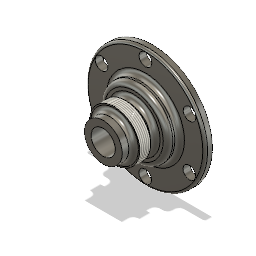
615789d2-998c-4c85-b917-ce7dc0a0639c (Autodesk Fusion 360 design; units mm, degrees)
Autodesk Fusion 360 part; units mm, degrees
sketch "Sketch1" plane through (0, 0, 0) normal (0, 0, 1) x (1, 0, 0)
  circle A0 centre (0, 0) radius 49.5
  dimension "d1" = 99
  measures "d1" diameter of A0
extrude "Extrude1" add sketch "Sketch1" along normal blind 6.1
sketch "Sketch2" plane through (0, 0, 6.1) normal (0, 0, 1) x (1, 0, 0)
  circle A0 centre (0, 0) radius 49.5
  circle A1 centre (0, 0) radius 42
  circle A2 centre (0, 42) radius 5.25
  circle A3 centre (-0.1888, -41.9996) radius 5.25
  line L0 (0, 0) -> (47.6946, 0) construction
  circle A4 centre (-36.3731, 21) radius 5.25
  circle A5 centre (-36.3731, -21) radius 5.25
  line L1 (0, 0) -> (42, 0) construction
  circle A6 centre (36.3731, -21) radius 5.25
  circle A7 centre (36.563, 21.1097) radius 5.25
  dimension "d4" = 84
  dimension "d5" = 10.5
  dimension "d7" = 10.5
  dimension "d11" = 10.5
  dimension "d12" = 10.5
  dimension "d15" = 10.5
  dimension "d16" = 10.5
  measures "d4" diameter of A1
  measures "d5" diameter of A2
  measures "d7" diameter of A3
  measures "d11" diameter of A4
  measures "d12" diameter of A5
  measures "d15" diameter of A6
  measures "d16" diameter of A7
extrude "Extrude2" cut sketch "Sketch2" against normal blind 15 contours A1 A7 | A1 A7 | A1 A6 | A1 A6 | A1 A2 | A1 A2 | A1 A3 | A1 A3 | A1 A4 | A1 A4 | A1 A5 | A1 A5
sketch "Sketch3" plane through (0, 0, 6.1) normal (0, 0, 1) x (1, 0, 0)
  circle A0 centre (36.3731, -21) radius 5.25
  circle A1 centre (-36.3731, 21) radius 5.25
  circle A2 centre (-0.1888, -41.9996) radius 5.25
  circle A3 centre (36.563, 21.1097) radius 5.25
  circle A4 centre (0, 42) radius 5.25
  circle A5 centre (-36.3731, -21) radius 5.25
  circle A6 centre (0, 0) radius 49.5
  circle A7 centre (0, 0) radius 28.3
  dimension "d19" = 56.6
  measures "d19" diameter of A7
extrude "Extrude3" add sketch "Sketch3" along normal blind 9.6 contours A7
sketch "Sketch4" plane through (0, 0, 0) normal (0, 0, -1) x (-1, 0, 0)
  circle A0 centre (-36.3731, -21) radius 5.25
  circle A1 centre (36.3731, 21) radius 5.25
  circle A2 centre (0.1888, -41.9996) radius 5.25
  circle A3 centre (-36.563, 21.1097) radius 5.25
  circle A4 centre (0, 42) radius 5.25
  circle A5 centre (36.3731, -21) radius 5.25
  circle A6 centre (0, 0) radius 49.5
  circle A7 centre (0, 0) radius 22.225
  dimension "d22" = 44.45
  measures "d22" diameter of A7
extrude "Extrude4" cut sketch "Sketch4" against normal blind 9.4 contours A7
sketch "Sketch5" plane through (0, 0, 15.7) normal (0, 0, 1) x (1, 0, 0)
  circle A0 centre (0, 0) radius 28.3
  circle A1 centre (0, 0) radius 17.75
  dimension "d25" = 35.5
  measures "d25" diameter of A1
extrude "Extrude5" add sketch "Sketch5" along normal blind 7 contours A1
sketch "Sketch6" plane through (0, 0, 22.7) normal (0, 0, 1) x (1, 0, 0)
  circle A0 centre (0, 0) radius 17.75
  circle A1 centre (0, 0) radius 21
  dimension "d28" = 42
  measures "d28" diameter of A1
extrude "Extrude6" add sketch "Sketch6" along normal blind 9 contours A0 | A1
thread "Thread1" "ANSI Metric M Profile 42.0 M42x1.5 6g" major diameter 41.85 minor diameter 40.1319 pitch 1.5 angle 60 resizes the face on face at (20.9739, -1.0468, 28.7)
sketch "Sketch7" plane through (0, 0, 31.7) normal (0, 0, 1) x (1, 0, 0)
  circle A0 centre (0, 0) radius 20.925
  circle A1 centre (0, 0) radius 15.8
  dimension "d31" = 31.6
  measures "d31" diameter of A1
extrude "Extrude7" add sketch "Sketch7" along normal blind 9.4 contours A1
sketch "Sketch8" plane through (0, 0, 41.1) normal (0, 0, 1) x (1, 0, 0)
  circle A0 centre (0, 0) radius 15.8
  circle A1 centre (0, 0) radius 10
  dimension "d34" = 20
  measures "d34" diameter of A1
extrude "Extrude8" cut sketch "Sketch8" against normal blind 31.7 contours A1
fillet "Fillet1" radius 2 1 edges at (-46.1502, -17.9, 6.1)
fillet "Fillet2" radius 4 4 edges at (-26.3849, 10.2337, 6.1) (-26.3849, -10.2337, 15.7) (-16.5488, 6.4187, 15.7) (-14.7308, 5.7135, 31.7)
fillet "Fillet3" radius 4 1 edges at (20.721, 8.0369, 9.4)
